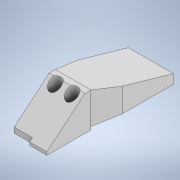
# Autodesk Inventor part: Finger_right_3
Saved by Autodesk Inventor 2022 (Build 260153000, 153)
## iProperties
Created: 2021-09-24
Part Number: Finger_right_3
Material: Generic
Document SubType Name: Modeling
Designer: kylem
Density: 1 g/cm^3
Appearance: Default
Author: kylem
Autodesk Inventor part; units mm, degrees
sketch "Sketch2" plane through (0, 0, 0) normal (0, 1, 0) x (-1, 0, 0)
  line L0 (0, 0) -> (19, 0)
  line L1 (19, 0) -> (19, 22)
  line L2 (19, 22) -> (0, 22)
  line L3 (0, 22) -> (0, 0)
  line L4 (19, 22) -> (14, 22)
  line L5 (14, 22) -> (14, 5)
  line L6 (14, 5) -> (19, 5)
  line L7 (19, 5) -> (19, 22)
  line L8 (0, 22) -> (5, 22)
  line L9 (5, 22) -> (5, 5)
  line L10 (5, 5) -> (0, 5)
  line L11 (0, 5) -> (0, 22)
  circle A0 centre (14, 5) radius 1.7
  circle A1 centre (5, 5) radius 1.7
  dimension "d0" = 19
  dimension "d1" = 22
  dimension "d2" = 5
  dimension "d3" = 17
  dimension "d4" = 5
  dimension "d5" = 17
  dimension "d6" = 3.4
  dimension "d7" = 3.4
  constraints: 24 end point, 6 parallel, 3 horizontal, 3 perpendicular, 2 centre point, 2 coincident
  measures "d0" distance of L2.end L1.end
  measures "d1" distance of L1.end L0.end
  measures "d2" distance of L6.end L5.end
  measures "d3" distance of L5.end L4.end
  measures "d4" distance of L9.end L10.end
  measures "d5" distance of L8.end L9.end
  measures "d6" diameter of A0
  measures "d7" diameter of A1
extrude "Extrusion1" add sketch "Sketch2" along normal blind 17.2 contours L3 L10 A1 L9 L2 L5 A0 L6 L1 L0 | L3 L2 L9 A1 L10 | L6 A0 L5 L2 L1
sketch "Sketch4" plane through (0, 0, 22) normal (1, 0, 0) x (0, 0, -1)
  line L0 (0, 0) -> (17.2, 0)
  line L1 (17.2, 0) -> (-6, 0)
  line L2 (-6, 0) -> (-6, -60)
  line L3 (-6, -60) -> (17.2, -60)
  line L4 (17.2, -60) -> (17.2, 0)
  line L5 (0, 0) -> (17.2, 0)
  line L6 (17.2, 0) -> (-6, 0)
  line L7 (-6, 0) -> (-6, -60)
  line L8 (-6, -60) -> (17.2, -60)
  line L9 (17.2, -60) -> (17.2, 0)
  line L10 (0, 0) -> (22, 0) projected
  line L11 (22, 0) -> (22, -6)
  line L12 (22, -6) -> (82, -6)
  line L13 (82, -6) -> (82, 17.2)
  line L14 (82, 17.2) -> (22, 17.2)
  line L15 (22, 17.2) -> (22, -6)
  point P0 (0, 22)
  point P1 (0, 22)
  dimension "d15" = 23.2
  dimension "d16" = 60
  dimension "d17" = 23.2
  dimension "d18" = 60
  dimension "d19" = 6
  dimension "d20" = 60
  dimension "d21" = 23.2
  constraints: 30 end point, 6 parallel, 3 horizontal, 3 perpendicular, 1 vertical
  measures "d15" distance of L3.end L2.end
  measures "d16" distance of L2.end L1.end
  measures "d17" distance of L8.end L7.end
  measures "d18" distance of L7.end L6.end
  measures "d19" distance of L10.end L11.end
  measures "d20" distance of L14.end L13.end
  measures "d21" distance of L13.end L12.end
extrude "Extrusion2" add sketch "Sketch4" against normal blind 19 contours L15 L14 L13 L12 L11
sketch "Sketch5" plane through (0, -6, -60) normal (0, -1, 0) x (1, 0, 0)
  line L0 (0, 82) -> (0, 0) projected
  line L1 (-19, 82) -> (-19, 0) projected
  line L2 (0, 0) -> (-19, 0)
  line L3 (-19, 0) -> (-19, 38.5)
  line L4 (-19, 38.5) -> (0, 38.5)
  line L5 (0, 38.5) -> (0, 0)
  point P0 (0, 60)
  dimension "d24" = 38.5
  constraints: 8 end point, 2 parallel, 1 horizontal, 1 perpendicular, 1 point on line
  measures "d24" distance of L2.end L3.end
extrude "Extrusion3" cut sketch "Sketch5" against normal blind 18.2
sketch "Sketch6" plane through (0, 17.2, 0) normal (0, 1, 0) x (1, 0, 0)
  line L0 (0, -22) -> (0, 0) projected
  line L1 (-19, 21.5) -> (-19, 0) projected
  line L2 (0, -22) -> (-19, -22)
  line L3 (-19, -22) -> (-19, 0)
  line L4 (-19, 0) -> (0, 0)
  line L5 (0, 0) -> (0, -22)
  dimension "d27" = 22
  constraints: 8 end point, 2 parallel, 1 horizontal, 1 perpendicular
  measures "d27" distance of L2.end L1.end
extrude "Extrusion4" cut sketch "Sketch6" against normal blind 10
sketch "Sketch7" plane through (0, 17.2, 0) normal (0, 1, 0) x (1, 0, 0)
  line L0 (0, -22) -> (0, 0) projected
  line L1 (0, 0) -> (-19, 0) projected
  line L2 (0, 0) -> (-19, 0)
  line L3 (-9.5, 0) -> (6.4, 0)
  line L4 (6.4, 0) -> (6.4, 21.5)
  line L5 (0, 0) -> (0, 21.5) projected
  line L6 (6.4, 21.5) -> (0, 21.5)
  line L7 (0, 21.5) -> (0, 0)
  line L8 (0, 0) -> (6.4, 0)
  line L9 (6.4, 0) -> (6.4, 21.5)
  line L10 (-19, 21.5) -> (-19, 0) projected
  line L11 (-9.5, 0) -> (-19, 0)
  line L12 (-19, 0) -> (-19, 21.5)
  line L13 (-19, 21.5) -> (-9.5, 21.5)
  line L14 (-9.5, 21.5) -> (-9.5, 0)
  line L15 (-9.5, 0) -> (-25.4, 0)
  line L16 (-25.4, 0) -> (-25.4, 21.5)
  line L17 (-25.4, 21.5) -> (-9.5, 21.5)
  line L18 (-9.5, 21.5) -> (-9.5, 0)
  line L19 (6.4, 21.5) -> (0, 0)
  line L20 (-25.4, 21.5) -> (-19, 0)
  dimension "d30" = 15.9
  dimension "d31" = 21.5
  dimension "d32" = 15.9
  constraints: 34 end point, 6 parallel, 4 horizontal, 3 perpendicular, 2 point on line, 1 midpoint, 1 vertical
  measures "d30" distance of L3.start L3.end
  measures "d31" distance of L3.end L4.end
  measures "d32" distance of L16.end L17.end
extrude "Extrusion5" add sketch "Sketch7" against normal blind 23.2 contours L5 L6 L19 | L20 L17 L10
sketch "Sketch8" plane through (0, 17.2, 0) normal (0, 1, 0) x (1, 0, 0)
  line L0 (6.4, 21.5) -> (0, 0) projected
  line L1 (0, 21.5) -> (0, 60) projected
  line L2 (6.4, 21.5) -> (0, 21.5)
  line L3 (0, 21.5) -> (0, 60)
  line L4 (0, 60) -> (6.4, 60)
  line L5 (6.4, 60) -> (6.4, 21.5)
  line L6 (-19, 60) -> (-19, 21.5) projected
  line L7 (-19, 0) -> (-25.4, 21.5) projected
  line L8 (-19, 60) -> (-25.4, 60)
  line L9 (-25.4, 60) -> (-25.4, 21.5)
  line L10 (-25.4, 21.5) -> (-19, 21.5)
  line L11 (-19, 21.5) -> (-19, 60)
  constraints: 16 end point, 4 parallel, 2 horizontal, 2 perpendicular
extrude "Extrusion6" add sketch "Sketch8" against normal blind 5
chamfer "Chamfer1" [suppressed]
ref_plane "Work Plane1" through (-25.4, 8, -21.5) normal (0, -1, 0) x (1, 0, 0)
chamfer "Chamfer4" distance 12 angle 25 1 edges at (-9.5, 7.2, 22) measured on face at (-10.7991, 7.2, 16.8632)
sketch "Sketch10" plane through (0, 12.2, -60) normal (0, -1, 0) x (1, 0, 0)
  line L0 (-25.4, 38.5) -> (6.4, 38.5)
  line L1 (-25.4, 38.5) -> (6.4, 38.5)
  line L2 (-9.5, 38.5) -> (-9.5, 26)
  line L3 (-9.5, 26) -> (-9.5, 6)
  line L4 (-9.5, 16) -> (-19.5, 16)
  line L5 (-19.5, 16) -> (0.5, 16)
  circle A0 centre (-19.5, 16) radius 1.7
  circle A1 centre (-9.5, 6) radius 1.7
  circle A2 centre (-9.5, 26) radius 1.7
  circle A3 centre (0.5, 16) radius 1.7
  point P0 (0, 60)
  point P1 (0, 60)
  dimension "d70" = 12.5
  dimension "d71" = 20
  dimension "d72" = 10
  dimension "d73" = 20
  dimension "d74" = 3.4
  dimension "d75" = 3.4
  dimension "d76" = 3.4
  dimension "d77" = 3.4
  constraints: 12 end point, 4 centre point, 4 coincident, 2 midpoint, 2 point on line, 1 collinear, 1 horizontal, 1 vertical
  measures "d70" distance of L2.start L2.end
  measures "d71" distance of L2.end L3.end
  measures "d72" distance of L4.start L4.end
  measures "d73" distance of L4.end L5.end
  measures "d74" diameter of A0
  measures "d75" diameter of A1
  measures "d76" diameter of A2
  measures "d77" diameter of A3
extrude "Extrusion9" cut sketch "Sketch10" against normal blind 10
sketch "Sketch11" plane through (0, 17.2, 0) normal (0, 1, 0) x (1, 0, 0)
  circle A0 centre (0.5, 44) radius 1.7 projected
  circle A1 centre (0.5, 44) radius 3.25
  circle A2 centre (-9.5, 54) radius 1.7 projected
  circle A3 centre (-9.5, 54) radius 3.25
  circle A4 centre (-19.5, 44) radius 1.7 projected
  circle A5 centre (-19.5, 44) radius 3.25
  circle A6 centre (-9.5, 34) radius 1.7 projected
  circle A7 centre (-9.5, 34) radius 3.25
  point P0 (0, 60)
  dimension "d84" = 6.5
  dimension "d85" = 6.5
  dimension "d86" = 6.5
  dimension "d87" = 6.5
  constraints: 4 centre point, 4 coincident
  measures "d84" diameter of A1
  measures "d85" diameter of A3
  measures "d86" diameter of A5
  measures "d87" diameter of A7
extrude "Extrusion10" cut sketch "Sketch11" against normal blind 3 contours A1 | A2 | A3 | A4 | A5 | A6 | A7
ref_plane "Work Plane2" through (-9.5, 17.2, -60) normal (-1, 0, 0) x (0, 0, 1)
chamfer "Chamfer6" [suppressed]
sketch "l" plane through (-19, 0, 0) normal (-1, 0, 0) x (0, 0, 1)
  line L0 (22, 1.6043) -> (10, 7.2) projected
  line L1 (10, 7.2) -> (32.2401, -3.1707)
  line L2 (0, 0) -> (22, 0) projected
  line L3 (0, 0) -> (30.1828, 0)
  line L4 (22, 0) -> (23.5, 0)
  line L5 (23.5, 0) -> (23.5, 4.1635)
  line L6 (22, 0) -> (22, 1.6043) projected
  line L7 (22, 1.6043) -> (22, 0)
  point P0 (23.5, 0.9048)
  dimension "d104" = 1.5
  constraints: 10 end point, 2 collinear, 1 horizontal, 1 perpendicular, 1 point on line
  measures "d104" distance of L2.end L4.end
extrude "Extrusion12" add sketch "l" against normal blind 9.2 contours L1 L5 L3 L6
sketch "Sketch14" plane through (-19, 0, 0) normal (-1, 0, 0) x (0, 0, 1)
  line L0 (0, 17.2) -> (25.44, 17.2)
  line L1 (25.44, 17.2) -> (25.44, 0)
  line L2 (25.44, 0) -> (0, 0)
  line L3 (0, 0) -> (0, 17.2)
  line L4 (0, 17.2) -> (25.44, 0)
  dimension "d107" = 25.44
  constraints: 10 end point, 2 parallel, 1 horizontal, 1 perpendicular
  measures "d107" distance of L1.end L2.end
extrude "Extrusion13" add sketch "Sketch14" against normal blind 19 contours L4 L2 L3
sketch "Sketch15" plane through (0, 0, 0) normal (0, -1, 0) x (1, 0, 0)
  line L0 (6.4, -21.5) -> (0, 0) projected
  line L1 (0, 0) -> (0, 5)
  line L2 (0, 25.44) -> (0, 0) projected
  line L3 (0, 5) -> (0, 10)
  line L4 (0, 5) -> (-5, 5)
  line L5 (0, 0) -> (-19, 0) projected
  line L6 (-19, 0) -> (-19, 5)
  line L7 (-19, 0) -> (-19, 25.44) projected
  line L8 (-19, 5) -> (-14, 5)
  circle A0 centre (-14, 5) radius 1.6
  circle A1 centre (-5, 5) radius 1.6
  point P0 (0.5177, -1.7393)
  point P1 (0.9, -3.0234)
  dimension "d110" = 5
  dimension "d111" = 5
  dimension "d112" = 5
  dimension "d113" = 5
  dimension "d114" = 5
  dimension "d115" = 3.2
  dimension "d116" = 3.2
  constraints: 10 end point, 3 point on line, 2 centre point, 2 coincident, 1 horizontal, 1 perpendicular
  measures "d110" distance of L0.end L1.end
  measures "d111" distance of L1.end L3.end
  measures "d112" distance of L1.end L4.end
  measures "d113" distance of L5.end L6.end
  measures "d114" distance of L6.end L8.end
  measures "d115" diameter of A0
  measures "d116" diameter of A1
extrude "Extrusion14" cut sketch "Sketch15" against normal blind 19
ref_plane "Work Plane3" through (0, 6.5, 0) normal (0, -1, 0) x (1, 0, 0)
sketch "Sketch16" plane through (0, 6.5, 0) normal (0, -1, 0) x (1, 0, 0)
  circle A0 centre (-14, 5) radius 1.6 projected
  circle A1 centre (-14, 5) radius 3
  circle A2 centre (-5, 5) radius 1.6 projected
  circle A3 centre (-5, 5) radius 3
  point P0 (0, 0)
  dimension "d120" = 6
  dimension "d121" = 6
  constraints: 2 centre point, 2 coincident
  measures "d120" diameter of A1
  measures "d121" diameter of A3
extrude "Extrusion15" cut sketch "Sketch16" against normal blind 19
sketch "Sketch17" plane through (0, 17.2, 0) normal (0, 1, 0) x (1, 0, 0)
  line L0 (6.4, 60) -> (-25.4, 60) projected
  line L1 (0, 0) -> (6.4, 21.5) projected
  line L2 (6.4, 60) -> (6.4, 21.5)
  line L3 (0, 0) -> (-19, 0) projected
  line L4 (6.4, 21.5) -> (0, 0)
  line L5 (0, 0) -> (-19, 0)
  line L6 (-19, 0) -> (-25.4, 21.5)
  line L7 (-25.4, 21.5) -> (-25.4, 60)
  line L8 (-25.4, 60) -> (6.4, 60)
  circle A0 centre (-9.5, 54) radius 3.25 projected
  circle A1 centre (-9.5, 54) radius 3.25
  circle A2 centre (0.5, 44) radius 1.7 projected
  circle A3 centre (0.5, 44) radius 3.25
  circle A4 centre (-9.5, 34) radius 1.7 projected
  circle A5 centre (-9.5, 34) radius 3.25
  circle A6 centre (-19.5, 44) radius 1.7 projected
  circle A7 centre (-19.5, 44) radius 3.25
  constraints: 12 end point, 4 centre point, 4 coincident, 2 equal length, 1 perpendicular, 1 vertical
extrude "Extrusion16" add sketch "Sketch17" along normal blind 4 contours L2 L1 L3 L6 L7 L0
sketch "Sketch18" plane through (-19, 0, 0) normal (-1, 0, 0) x (0, 0, 1)
  line L0 (0, 21.2) -> (25.44, 0)
  line L1 (25.44, 0) -> (0, 17.2)
  line L2 (0, 17.2) -> (0, 21.2) projected
  line L3 (0, 17.2) -> (0, 21.2)
  point P0 (0, 0)
  constraints: 6 end point, 1 collinear
extrude "Extrusion17" add sketch "Sketch18" against normal blind 19
extrude "Extrusion18" cut sketch "Sketch16" against normal blind 19 contours A0 | A1 | A2 | A3
sketch "Sketch20" plane through (0, 0, 25.44) normal (1, 0, 0) x (0, 0, -1)
  line L0 (25.44, 0) -> (0, 0) projected
  line L1 (0, 0) -> (1.94, 0)
  line L2 (1.94, 0) -> (1.94, 2.92)
  line L3 (1.94, 2.92) -> (0, 2.92)
  line L4 (0, 2.92) -> (0, 0)
  point P0 (1.94, 0)
  dimension "d148" = 1.94
  constraints: 8 end point, 2 parallel, 1 horizontal, 1 perpendicular
  measures "d148" distance of L3.end L2.end
extrude "Extrusion19" cut sketch "Sketch20" against normal blind 9.2
sketch "Sketch21" plane through (-19, 0, 0) normal (-1, 0, 0) x (0, 0, 1)
  line L0 (25.44, 0) -> (0, 21.2) projected
  line L1 (25.44, 0) -> (22, 0)
  line L2 (22, 0) -> (22, 4.8404)
  line L3 (22, 4.8404) -> (25.44, 4.8404)
  line L4 (25.44, 4.8404) -> (25.44, 0)
  point P0 (0, 0)
  point P1 (16.0198, 7.8502)
  dimension "d151" = 3.44
  constraints: 8 end point, 2 parallel, 1 horizontal, 1 perpendicular
  measures "d151" distance of L2.end L3.end
extrude "Extrusion20" cut sketch "Sketch21" against normal blind 9.8
sketch "Sketch22" plane through (-25.4, -6, -21.5) normal (0, -1, 0) x (1, 0, 0)
  line L0 (0, 0) -> (6.4, 21.5)
  line L1 (25.4, 21.5) -> (6.4, 21.5) projected
  line L2 (6.4, 21.5) -> (25.4, 21.5)
  line L3 (25.4, 21.5) -> (31.8, 0)
  line L4 (6.4, 21.5) -> (0, 0) projected
  line L5 (31.8, 0) -> (0, 0)
  constraints: 8 end point, 1 collinear, 1 parallel
extrude "Extrusion21" cut sketch "Sketch22" against normal blind 7.6
sketch "Sketch23" plane through (-25.4, 1.6, -21.5) normal (0, -1, 0) x (1, 0, 0)
  line L0 (0, 0) -> (6.4, 21.5) projected
  line L1 (6.4, 21.5) -> (-4.398, 21.5)
  line L2 (-4.398, 21.5) -> (-4.398, -43.3957)
  line L3 (-4.398, -43.3957) -> (6.4, -43.3957)
  line L4 (6.4, -43.3957) -> (6.4, 21.5)
  line L5 (25.4, 21.5) -> (31.8, 0) projected
  line L6 (25.4, 21.5) -> (33.9316, 21.5)
  line L7 (33.9316, 21.5) -> (33.9316, -42.1701)
  line L8 (33.9316, -42.1701) -> (25.4, -42.1701)
  line L9 (25.4, -42.1701) -> (25.4, 21.5)
  line L10 (0, 0) -> (31.8, 0) projected
  line L11 (31.8, -38.5) -> (0, -38.5) projected
  line L12 (0, 0) -> (31.8, 0)
  line L13 (31.8, 0) -> (31.8, -38.5)
  line L14 (31.8, -38.5) -> (0, -38.5)
  line L15 (0, -38.5) -> (0, 0)
  point P0 (0, -38.5)
  point P1 (25.4, 0)
  point P2 (6.4, 0)
  constraints: 24 end point, 6 parallel, 3 horizontal, 3 perpendicular
extrude "Extrusion22" cut sketch "Sketch23" against normal blind 40 contours L0 L4 L10 | L10 L4 L11 L15 | L10 L9 L11 L4 | L10 L13 L11 L9 | L9 L5 L10
sketch "Sketch25" plane through (0, 21.2, 0) normal (0, 1, 0) x (1, 0, 0)
  line L0 (8.5307, 32.4307) -> (-26.8903, 32.4307)
  line L1 (-26.8903, 32.4307) -> (-26.8903, -40.3587)
  line L2 (-26.8903, -40.3587) -> (8.5307, -40.3587)
  line L3 (8.5307, -40.3587) -> (8.5307, 32.4307)
  point P0 (0, 0)
  constraints: 8 end point, 2 parallel, 1 horizontal, 1 perpendicular
extrude "Extrusion23" cut sketch "Sketch25" against normal blind 14.7
sketch "Sketch26" plane through (0, 6.5, -21.5) normal (0, 0, -1) x (-1, 0, 0)
  line L0 (0, -4.9) -> (19, -4.9) projected
  line L1 (19, -3.6333) -> (19, 0) projected
  line L2 (0, -4.9) -> (19, -4.9)
  line L3 (19, -4.9) -> (19, 0)
  line L4 (19, 0) -> (0, 0)
  line L5 (0, 0) -> (0, -4.9)
  point P0 (0, -6.5)
  constraints: 8 end point, 2 parallel, 1 horizontal, 1 perpendicular
extrude "Extrusion24" add sketch "Sketch26" along normal blind 20
sketch "Sketch27" plane through (-25.4, 1.6, -21.5) normal (0, -1, 0) x (1, 0, 0)
  line L0 (6.4, 39.14) -> (6.4, -20) projected
  line L1 (6.4, -20) -> (3.9, -20)
  line L2 (3.9, -20) -> (3.9, 21.5)
  line L3 (3.9, 21.5) -> (6.4, 21.5)
  line L4 (6.4, 21.5) -> (6.4, -20)
  line L5 (25.4, 45) -> (25.4, 21.5) projected
  line L6 (25.4, 21.5) -> (27.9, 21.5)
  line L7 (27.9, 21.5) -> (27.9, -20)
  line L8 (27.9, -20) -> (25.4, -20)
  line L9 (25.4, -20) -> (25.4, 21.5)
  point P0 (6.4, 21.5)
  dimension "d165" = 2.5
  dimension "d166" = 2.5
  constraints: 16 end point, 4 parallel, 2 horizontal, 2 perpendicular, 1 point on line
  measures "d165" distance of L2.end L3.end
  measures "d166" distance of L7.end L8.end
extrude "Extrusion25" add sketch "Sketch27" against normal blind 4.9
sketch "Sketch28" plane through (-25.4, 1.6, -21.5) normal (0, -1, 0) x (1, 0, 0)
  line L0 (6.4, 39.14) -> (6.4, 21.5) projected
  line L1 (6.4, 21.5) -> (6.4, 7.3)
  line L2 (6.4, 7.3) -> (2.4289, 7.3)
  line L3 (3.9, -20) -> (3.9, 21.5) projected
  line L4 (6.4, 21.5) -> (25.4, 21.5) projected
  line L5 (3.9, 7.3) -> (6.4, 21.5)
  line L6 (3.9, 21.5) -> (6.4, 21.5)
  line L7 (6.4, 21.5) -> (6.4, 7.3)
  line L8 (6.4, 7.3) -> (3.9, 7.3)
  line L9 (3.9, 7.3) -> (3.9, 21.5)
  line L10 (15.9, 21.5) -> (15.9, 25.242)
  line L11 (15.9, 25.242) -> (15.9, 16.8089)
  line L12 (25.4, 39.14) -> (25.4, 21.5)
  line L13 (25.4, 21.5) -> (25.4, 7.3)
  line L14 (25.4, 7.3) -> (29.3711, 7.3)
  line L15 (27.9, -20) -> (27.9, 21.5)
  line L16 (25.4, 21.5) -> (6.4, 21.5)
  line L17 (27.9, 7.3) -> (25.4, 21.5)
  line L18 (27.9, 21.5) -> (25.4, 21.5)
  line L19 (25.4, 21.5) -> (25.4, 7.3)
  line L20 (25.4, 7.3) -> (27.9, 7.3)
  line L21 (27.9, 7.3) -> (27.9, 21.5)
  point P0 (6.4, 21.5)
  dimension "d169" = 14.2
  constraints: 38 end point, 10 symmetric about line, 5 point on line, 2 parallel, 2 perpendicular, 2 vertical, 1 horizontal, 1 midpoint
  measures "d169" distance of L0.end L1.end
extrude "Extrusion26" cut sketch "Sketch28" against normal blind 10 contours L18 L15 L17 | L5 L3 L6
sketch "Sketch29" plane through (0, 6.5, 0) normal (0, 1, 0) x (1, 0, 0)
  line L0 (-19, -22) -> (-19, -17.64) projected
  line L1 (-19, 0) -> (-19, -22) projected
  line L2 (-19, -17.64) -> (-19, 0)
  line L3 (-21.5, 14.2) -> (-21.5, 41.5) projected
  line L4 (-19, 0) -> (-21.5, 14.2)
  line L5 (-21.5, 14.2) -> (-21.5, 41.5)
  line L6 (2.5, 41.5) -> (-21.5, 41.5) projected
  line L7 (-21.5, 41.5) -> (2.5, 41.5)
  line L8 (2.5, 14.2) -> (2.5, 41.5) projected
  line L9 (2.5, 41.5) -> (2.5, 14.2)
  line L10 (2.5, 14.2) -> (0, 0)
  line L11 (0, -17.64) -> (-19, -17.64) projected
  line L12 (0, 0) -> (0, -17.64)
  line L13 (0, -17.64) -> (-19, -17.64)
  circle A0 centre (-14, -5) radius 1.6 projected
  circle A1 centre (-14, -5) radius 3
  circle A2 centre (-5, -5) radius 1.6 projected
  circle A3 centre (-5, -5) radius 3
  dimension "d172" = 6
  dimension "d173" = 6
  constraints: 16 end point, 3 perpendicular, 2 centre point, 2 coincident, 2 collinear, 1 vertical
  measures "d172" diameter of A1
  measures "d173" diameter of A3
extrude "Extrusion27" add sketch "Sketch29" along normal blind 12 contours L4 L3 L6 L8 L10 L12 L11 L1
sketch "Sketch30" plane through (-19, 0, 22) normal (-1, 0, 0) x (0, 0, 1)
  line L0 (-4.36, 6.5) -> (1.5, 1.6167) projected
  line L1 (1.5, 1.6167) -> (-4.36, 6.5)
  line L2 (-4.36, 6.5) -> (-25.2198, 23.8832)
  line L3 (-25.2198, 23.8832) -> (-1.43, 23.8832)
  line L4 (-14, 18.5) -> (-14, 6.5) projected
  line L5 (-1.43, 23.8832) -> (-4.36, 6.5)
  point P0 (-22, 0)
  dimension "d176" = 180
  constraints: 8 end point, 1 collinear, 1 perpendicular
  measures "d176" angle of L1 L2
extrude "Extrusion28" cut sketch "Sketch30" along normal mid plane 50
sketch "Sketch31" plane through (-19, 0, 22) normal (-1, 0, 0) x (0, 0, 1)
  line L0 (-22, 1.6) -> (-22, 18.5) projected
  line L1 (-36.2, 1.6) -> (-63.5, 1.6) projected
  line L2 (-22, 1.6) -> (-63.5, 1.6)
  line L3 (-63.5, 1.6) -> (-63.5, 6.6)
  line L4 (-63.5, 1.6) -> (-63.5, 18.5) projected
  line L5 (-22, 18.5) -> (-22, 1.6) projected
  line L6 (-63.5, 6.6) -> (-22, 18.5)
  line L7 (-22, 18.5) -> (-22, 1.6)
  line L8 (-63.5, 6.6) -> (-22, 18.5)
  line L9 (-22, 18.5) -> (-18.76, 18.5) projected
  line L10 (-63.5, 18.5) -> (-22, 18.5)
  line L11 (-63.5, 18.5) -> (-36.2, 18.5) projected
  line L12 (-22, 18.5) -> (-63.5, 18.5)
  line L13 (-63.5, 18.5) -> (-63.5, 6.6)
  point P0 (-22, 0)
  dimension "d179" = 5
  constraints: 16 end point, 4 collinear, 2 horizontal, 1 point on line
  measures "d179" distance of L1.end L3.end
extrude "Extrusion29" cut sketch "Sketch31" along normal mid plane 50 contours L6 L4 L10
body "Solid1"
